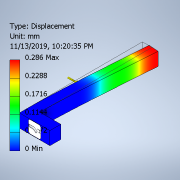
# Autodesk Inventor part: StressAnalysis
Saved by Autodesk Inventor 2020.1 (Build 241239000, 239)
## iProperties
Created: 2019-11-14
Part Number: StressAnalysis
Material: Balsa Wood
Document SubType Name: Modeling
Designer: super
Density: 0.166079 g/cm^3
Appearance: Generic
Author: super
Autodesk Inventor part; units mm, degrees
ref_plane "YZ Plane" through (0, 0, 0) normal (1, 0, 0) x (0, 1, 0)
ref_plane "XZ Plane" through (0, 0, 0) normal (0, 1, 0) x (-1, 0, 0)
ref_plane "XY Plane" through (0, 0, 0) normal (0, 0, 1) x (1, 0, 0)
sketch "Sketch1" plane through (0, 0, 0) normal (0, 1, 0) x (-1, 0, 0)
  line L0 (4.6687, 18.5347) -> (223.9143, 18.5347)
  line L1 (223.9143, 18.5347) -> (223.9143, 2837.3925)
  line L2 (223.9143, 2837.3925) -> (4.6687, 2837.3925)
  line L3 (4.6687, 2837.3925) -> (4.6687, 18.5347)
  point P0 (0, 0)
  constraints: 8 end point, 2 parallel, 1 horizontal, 1 perpendicular
extrude "Extrusion1" add sketch "Sketch1" against normal blind 300
sketch "Sketch2" plane through (-223.9143, 0, 18.5347) normal (-1, 0, 0) x (0, 0, -1)
  line L0 (-2818.8578, 0) -> (0, 0) projected
  line L1 (0, 300) -> (-2818.8578, 300) projected
  line L2 (0, 0) -> (250, 0)
  line L3 (250, 0) -> (250, 300)
  line L4 (250, 300) -> (0, 300)
  line L5 (0, 300) -> (0, 0)
  point P0 (18.5347, 0)
  point P1 (0, 300)
  dimension "d2" = 250
  constraints: 8 end point, 2 parallel, 1 horizontal, 1 perpendicular, 1 point on line
  measures "d2" distance of L4.end L3.end
extrude "Extrusion2" [suppressed]
sketch "Sketch3" plane through (-223.9143, 0, 2837.3925) normal (-1, 0, 0) x (0, 0, 1)
  line L0 (0, 0) -> (-2818.8578, 0) projected
  line L1 (-2818.8578, -300) -> (0, -300) projected
  line L2 (0, 0) -> (-250, 0)
  line L3 (-250, 0) -> (-250, -300)
  line L4 (-250, -300) -> (0, -300)
  line L5 (0, -300) -> (0, 0)
  point P0 (-2837.3925, 0)
  point P1 (0, -300)
  dimension "d5" = 250
  constraints: 8 end point, 2 parallel, 1 horizontal, 1 perpendicular, 1 point on line
  measures "d5" distance of L3.end L4.end
extrude "Extrusion3" add sketch "Sketch3" against normal blind 700
sketch "Sketch4" plane through (476.0857, 0, 2837.3925) normal (1, 0, 0) x (0, 0, 1)
  point P0 (-2837.3925, 0)
body "Solid1"
